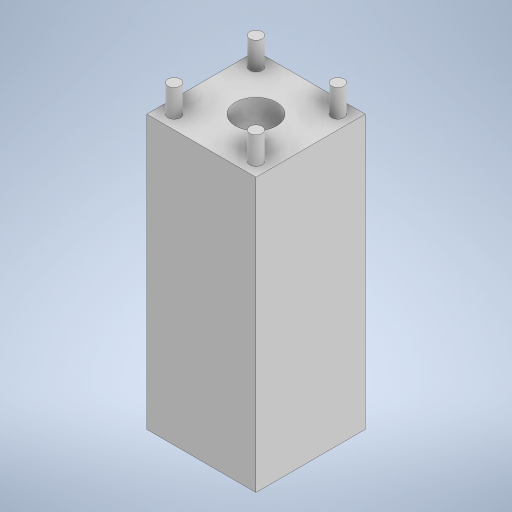
# Autodesk Inventor part: SpringAttachment
Saved by Autodesk Inventor 2024 (Build 280153000, 153)
## iProperties
Created: 2025-02-03
Part Number: SpringAttachment
Material: Generic
Document SubType Name: Modeling
Designer: matsk
Density: 1 g/cm^3
Appearance: Default
Author: matsk
Autodesk Inventor part; units mm, degrees
ref_plane "YZ Plane" through (0, 0, 0) normal (1, 0, 0) x (0, 1, 0)
ref_plane "XZ Plane" through (0, 0, 0) normal (0, 1, 0) x (-1, 0, 0)
ref_plane "XY Plane" through (0, 0, 0) normal (0, 0, 1) x (1, 0, 0)
sketch "Sketch1" plane through (0, 0, 0) normal (0, 1, 0) x (-1, 0, 0)
  line L0 (2, 2) -> (-2, 2)
  line L1 (-2, 2) -> (-2, -2)
  line L2 (-2, -2) -> (2, -2)
  line L3 (2, -2) -> (2, 2)
  line L4 (2, 2) -> (-2, -2) construction
  line L5 (-2, 2) -> (2, -2) construction
  circle A0 centre (0, 0) radius 0.75
  dimension "d0" = 4
  dimension "d1" = 4
  dimension "d2" = 1.5
  constraints: 12 end point, 2 midpoint, 2 parallel, 1 centre point, 1 coincident, 1 horizontal, 1 perpendicular
  measures "d0" distance of L2.end L1.end
  measures "d1" distance of L1.end L0.end
  measures "d2" diameter of A0
extrude "Extrusion1" add sketch "Sketch1" along normal blind 10
sketch "Sketch2" plane through (0, 10, 0) normal (0, 1, 0) x (1, 0, 0)
  line L0 (-1.5, 1.5) -> (1.5, -1.5) construction
  line L1 (1.5, 1.5) -> (-1.5, -1.5) construction
  circle A0 centre (1.5, -1.5) radius 0.225
  circle A1 centre (1.5, 1.5) radius 0.225
  circle A2 centre (-1.5, 1.5) radius 0.225
  circle A3 centre (-1.5, -1.5) radius 0.225
  point P0 (0, 0)
  dimension "d5" = 3
  dimension "d7" = 0.45
  dimension "d8" = 0.45
  dimension "d9" = 0.45
  dimension "d10" = 0.45
  constraints: 4 centre point, 4 end point, 2 coincident, 2 midpoint
  measures "d5" distance of L0.end L1.end
  measures "d7" diameter of A0
  measures "d8" diameter of A1
  measures "d9" diameter of A2
  measures "d10" diameter of A3
extrude "Extrusion2" add sketch "Sketch2" along normal blind 1
sketch "Sketch3" plane through (0, 0, 0) normal (0, -1, 0) x (1, 0, 0)
  line L0 (1, 0.25) -> (-1, 0.25)
  line L1 (-1, 0.25) -> (-1, -0.25)
  line L2 (-1, -0.25) -> (1, -0.25)
  line L3 (1, -0.25) -> (1, 0.25)
  line L4 (1, 0.25) -> (-1, -0.25) construction
  line L5 (-1, 0.25) -> (1, -0.25) construction
  point P0 (0, 0)
  dimension "d13" = 2
  dimension "d14" = 0.5
  constraints: 12 end point, 2 midpoint, 2 parallel, 1 horizontal, 1 perpendicular
  measures "d13" distance of L2.end L1.end
  measures "d14" distance of L1.end L0.end
extrude "Extrusion3" add sketch "Sketch3" against normal blind 0.5
fillet "Fillet1" radius 0.25 4 edges at (0, 0, 0.25) (0, 0, -0.25) (0, 0.5, 0.25) (0, 0.5, -0.25)
body "Solid1"
